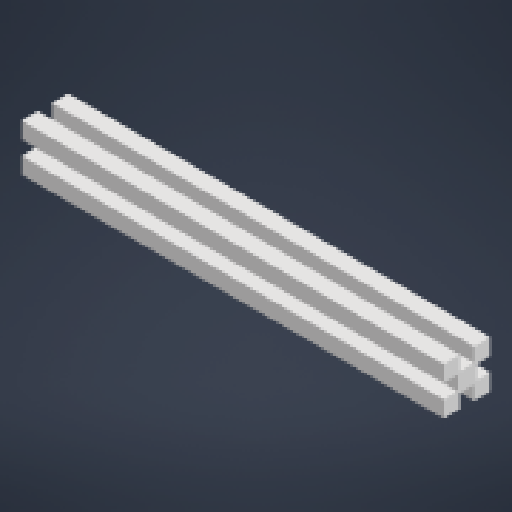
# Autodesk Inventor part: ybar
Saved by Autodesk Inventor 2025.1 (Build 291241020, 241B)
## iProperties
Created: 2024-09-23
Part Number: ybar
Material: Generic
Document SubType Name: Modeling
Designer: techn
Density: 1 g/cm^3
Appearance: Default
Author: techn
Autodesk Inventor part; units mm, degrees
ref_plane "YZ Plane" through (0, 0, 0) normal (1, 0, 0) x (0, 1, 0)
ref_plane "XZ Plane" through (0, 0, 0) normal (0, 1, 0) x (-1, 0, 0)
ref_plane "XY Plane" through (0, 0, 0) normal (0, 0, 1) x (1, 0, 0)
sketch "Sketch1" plane through (0, 0, 0) normal (1, 0, 0) x (0, 1, 0)
  line L0 (-8.5, -445) -> (-8.5, -5) projected
  line L1 (11.5, -5) -> (11.5, -445) projected
  line L2 (-8.5, -5) -> (-1.5, -5)
  line L3 (-1.5, -5) -> (-1.5, 2)
  line L4 (-1.5, 2) -> (-8.5, 2)
  line L5 (-8.5, 2) -> (-8.5, -5)
  line L6 (11.5, -5) -> (4.5, -5)
  line L7 (4.5, -5) -> (4.5, 2)
  line L8 (4.5, 2) -> (11.5, 2)
  line L9 (11.5, 2) -> (11.5, -5)
  line L10 (11.5, 8) -> (4.5, 8)
  line L11 (4.5, 8) -> (4.5, 15)
  line L12 (4.5, 15) -> (11.5, 15)
  line L13 (11.5, 15) -> (11.5, 8)
  line L14 (-8.5, 8) -> (-1.5, 8)
  line L15 (-1.5, 8) -> (-1.5, 15)
  line L16 (-1.5, 15) -> (-8.5, 15)
  line L17 (-8.5, 15) -> (-8.5, 8)
  line L18 (5.5, 1) -> (-2.5, 1)
  line L19 (-2.5, 1) -> (-2.5, 9)
  line L20 (-2.5, 9) -> (5.5, 9)
  line L21 (5.5, 9) -> (5.5, 1)
  point P0 (0, 0)
  point P1 (5.5, 2)
  point P2 (5.5, 8)
  point P3 (4.5, 9)
  point P4 (-1.5, 9)
  point P5 (-2.5, 8)
  point P6 (-2.5, 2)
  point P7 (-1.5, 1)
  point P8 (4.5, 1)
  dimension "d0" = 7
  dimension "d1" = 7
  dimension "d2" = 7
  dimension "d3" = 7
  dimension "d4" = 7
  dimension "d5" = 7
  dimension "d6" = 7
  dimension "d7" = 7
  dimension "d8" = 6
  dimension "d9" = 8
  dimension "d10" = 8
  dimension "d11" = 1
  dimension "d12" = 1
  constraints: 40 end point, 10 parallel, 5 horizontal, 5 perpendicular, 3 point on line
  measures "d0" distance of L4.end L3.end
  measures "d1" distance of L3.end L2.end
  measures "d2" distance of L7.end L8.end
  measures "d3" distance of L6.end L7.end
  measures "d4" distance of L11.end L12.end
  measures "d5" distance of L10.end L11.end
  measures "d6" distance of L16.end L15.end
  measures "d7" distance of L15.end L14.end
  measures "d8" distance between parallel lines of L4 L14
  measures "d9" distance of L19.end L20.end
  measures "d10" distance of L18.end L19.end
  measures "d11" distance between parallel lines of L18 L8
  measures "d12" distance between parallel lines of L7 L21
extrude "Extrusion1" add sketch "Sketch1" along normal blind 162 and the other way blind 18
body "Solid1"
